Autodesk Fusion 360 part; units mm, degrees
(part 4 of 5)
equation "d178 = ( 7.087 / 2 ) * 1 mm + 2 mm"
equation "d179 = ( 7.087 / 2 ) * 1 mm + 2 mm"
equation "d208 = ( 36.1 / 2 ) * 1 mm"
equation "d215 = ( 4.85 / 2 ) * 1 mm + 2 mm"
equation "d216 = ( 4.85 / 2 ) * 1 mm + 2 mm"
equation "d221 = ( 4.85 / 2 ) * 1 mm + 2 mm"
equation "d222 = ( 4.85 / 2 ) * 1 mm + 2 mm"
equation "d230 = ( 36.1 / 2 ) * 1 mm"
equation "d251 = ( 11.15 / 2 ) * 1 mm"
equation "d266 = ( 11.15 / 2 ) * 1 mm"

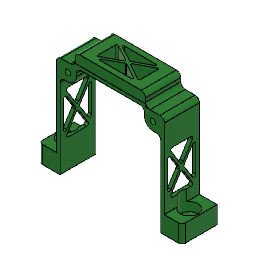
design "TM Front Holder"
Autodesk Fusion 360 part; units mm, degrees
sketch "Sketch1" plane through (0, 0, 0) normal (0, 0, 1) x (1, 0, 0)
  line L0 (28.55, 26.275) -> (30.55, 26.275)
  line L1 (30.55, 26.275) -> (30.55, -30.825)
  line L2 (30.55, -30.825) -> (28.55, -30.825)
  line L3 (28.55, -30.825) -> (28.55, 26.275)
  line L4 (-28.55, -30.825) -> (-30.55, -30.825)
  line L5 (-28.55, 26.275) -> (-28.55, -30.825)
  line L6 (-30.55, -30.825) -> (-30.55, 26.275)
  line L7 (-30.55, 26.275) -> (-28.55, 26.275)
  line L8 (-30.55, 26.275) -> (30.55, 26.275)
  line L9 (30.55, 26.275) -> (30.55, 28.275)
  line L10 (30.55, 28.275) -> (-30.55, 28.275)
  line L11 (-30.55, 28.275) -> (-30.55, 26.275)
  dimension "d1" = 2
  dimension "d4" = 26.275
  dimension "d5" = 2
  dimension "d7" = 57.1
  dimension "d8" = 28.55
  dimension "d9" = 2
  dimension "d99" = 59.1
  constraint horizontal L0
  constraint vertical L1
  constraint horizontal L2
  constraint vertical L3
  constraint horizontal L7
  constraint vertical L5
  constraint horizontal L4
  constraint vertical L6
  constraint horizontal L2.end L4.start
  constraint horizontal L8
  constraint vertical L9
  constraint horizontal L10
  constraint vertical L11
  constraint vertical L0.end L9.end
  measures "d1" distance of L1 L3
  measures "d4" distance of origin L0
  measures "d5" distance of L5 L6
  measures "d7" distance of L3 L5
  measures "d8" distance of origin L5
  measures "d9" distance of L8 L10
  measures "d99" distance of L2 L10
extrude "Extrude1" add sketch "Sketch1" along normal blind 20
sketch "Sketch2" plane through (0, 0, 20) normal (0, 0, 1) x (-1, 0, 0)
  line L0 (-30.55, 30.825) -> (-30.55, -28.275)
  line L1 (-30.55, -28.275) -> (30.55, -28.275)
  line L2 (30.55, -28.275) -> (30.55, 30.825)
  line L3 (30.55, 30.825) -> (28.55, 30.825)
  line L4 (28.55, 30.825) -> (28.55, -26.275)
  line L5 (28.55, -26.275) -> (-28.55, -26.275)
  line L6 (-28.55, -26.275) -> (-28.55, 30.825)
  line L7 (-28.55, 30.825) -> (-30.55, 30.825)
  line L8 (-30.55, 30.825) -> (-40.55, 30.825)
  line L9 (-40.55, 30.825) -> (-40.55, 28.325)
  line L10 (-40.55, 28.325) -> (-30.55, 28.325)
  line L11 (-30.55, 28.325) -> (-30.55, 30.825)
  line L12 (30.55, 30.825) -> (40.55, 30.825)
  line L13 (40.55, 30.825) -> (40.55, 28.325)
  line L14 (40.55, 28.325) -> (30.55, 28.325)
  line L15 (30.55, 28.325) -> (30.55, 30.825)
  dimension "d12" = 2.5
  dimension "d13" = 10
  dimension "d14" = 2.5
  dimension "d15" = 10
  constraint horizontal L8
  constraint vertical L9
  constraint horizontal L10
  constraint vertical L11
  constraint coincident L0.start L7.end
  constraint horizontal L12
  constraint vertical L13
  constraint horizontal L14
  constraint vertical L15
  constraint coincident L2.end L3.start
  measures "d12" distance of L8 L10
  measures "d13" distance of L9 L11
  measures "d14" distance of L12 L14
  measures "d15" distance of L13 L15
extrude "Extrude2" add sketch "Sketch2" against normal blind 20 contours L0 L8 L9 L10 L11 | L2 L12 L13 L14 L15
sketch "Sketch5" plane through (0, 28.275, 0) normal (0, 1, 0) x (-1, 0, 0)
  line L0 (-30.55, 0) -> (30.55, 0)
  line L1 (30.55, 0) -> (30.55, 20)
  line L2 (30.55, 20) -> (-30.55, 20)
  line L3 (-30.55, 20) -> (-30.55, 0)
  line L4 (-20, 20) -> (20, 20)
  line L5 (20, 20) -> (20, 0)
  line L6 (20, 0) -> (-20, 0)
  line L7 (-20, 0) -> (-20, 20)
  dimension "d32" = 40
  dimension "d96" = 20
  constraint horizontal L4
  constraint vertical L5
  constraint horizontal L6
  constraint vertical L7
  constraint coincident L0 L5.end
  constraint coincident L2 L4.start
  measures "d32" distance of L5 L7
  measures "d96" distance of origin L7
extrude "Extrude4" add sketch "Sketch5" along normal blind 10 contours L0 L2 L4 L5 L6 L7
sketch "Sketch6" plane through (0, 0, 0) normal (0, 0, -1) x (1, 0, 0)
  line L0 (20, -38.275) -> (20, -28.275)
  line L1 (-30.55, -28.275) -> (-20, -28.275)
  line L2 (30.55, -28.275) -> (30.55, 28.325)
  line L3 (30.55, 28.325) -> (40.55, 28.325)
  line L4 (40.55, 30.825) -> (28.55, 30.825)
  line L5 (28.55, 30.825) -> (28.55, -26.275)
  line L6 (28.55, -26.275) -> (-28.55, -26.275)
  line L7 (-28.55, -26.275) -> (-28.55, 30.825)
  line L8 (-28.55, 30.825) -> (-40.55, 30.825)
  line L9 (-40.55, 28.325) -> (-30.55, 28.325)
  line L10 (-30.55, 28.325) -> (-30.55, -28.275)
  line L11 (-20, -28.275) -> (-20, -38.275)
  line L12 (-20, -38.275) -> (20, -38.275)
  line L13 (-28.55, -26.275) -> (-19.3, -26.275)
  line L14 (-19.3, -23.775) -> (-19.3, -22.025)
  line L15 (-24.3, -17.025) -> (-26.05, -17.025)
  line L16 (-28.55, -17.025) -> (-28.55, -26.275)
  line L17 (28.55, -26.275) -> (19.3, -26.275)
  line L18 (19.3, -23.775) -> (19.3, -22.025)
  line L19 (24.3, -17.025) -> (26.05, -17.025)
  line L20 (28.55, -17.025) -> (28.55, -26.275)
  arc A0 (-19.3, -22.025) -> (-24.3, -17.025) centre (-24.3, -22.025) ccw
  arc A1 (24.3, -17.025) -> (19.3, -22.025) centre (24.3, -22.025) ccw
  line L21 (28.55, -14.525) -> (28.55, -10)
  line L22 (-28.55, -14.525) -> (-28.55, -10)
  arc A2 (26.05, -17.025) -> (28.55, -14.525) centre (26.05, -14.525) ccw
  arc A3 (-28.55, -14.525) -> (-26.05, -17.025) centre (-26.05, -14.525) ccw
  line L23 (16.8, -26.275) -> (13, -26.275)
  line L24 (-16.8, -26.275) -> (-13, -26.275)
  arc A4 (16.8, -26.275) -> (19.3, -23.775) centre (16.8, -23.775) ccw
  arc A5 (-19.3, -23.775) -> (-16.8, -26.275) centre (-16.8, -23.775) ccw
  line L25 (20, -28.275) -> (30.55, -28.275)
  line L26 (-40.55, 30.825) -> (-40.55, 28.325)
  line L27 (40.55, 28.325) -> (40.55, 30.825)
  dimension "d38" = 9.25
  dimension "d39" = 9.25
  dimension "d40" = 9.25
  dimension "d41" = 9.25
  dimension "d42" = 5
  dimension "d43" = 5
  dimension "d44" = 2.5
  dimension "d45" = 2.5
  dimension "d46" = 2.5
  dimension "d47" = 2.5
  constraint horizontal L13
  constraint vertical L14
  constraint horizontal L15
  constraint vertical L16
  constraint coincident L6.end L7.start
  constraint horizontal L17
  constraint vertical L18
  constraint horizontal L19
  constraint vertical L20
  constraint coincident L5.end L6.start
  constraint tangent L15 A0
  constraint tangent L14 A0
  constraint tangent L19 A1
  constraint tangent L18 A1
  constraint coincident L5 L21.end
  constraint coincident L7 L22.end
  constraint coincident L20.start L19
  constraint coincident L20.start L21
  constraint tangent L19 A2
  constraint tangent L21 A2
  constraint coincident L16.start L22
  constraint coincident L16.start L15
  constraint tangent L22 A3
  constraint tangent L15 A3
  constraint coincident L6 L23.end
  constraint coincident L6 L24.end
  constraint coincident L17.end L23
  constraint coincident L17.end L18
  constraint tangent L23 A4
  constraint tangent L18 A4
  constraint coincident L13.end L24
  constraint coincident L13.end L14
  constraint tangent L24 A5
  constraint tangent L14 A5
  measures "d38" distance of L14 L16
  measures "d39" distance of L13 L15
  measures "d40" distance of L18 L20
  measures "d41" distance of L17 L19
  measures "d42" radius of A0
  measures "d43" radius of A1
  measures "d44" radius of A2
  measures "d45" radius of A3
  measures "d46" radius of A4
  measures "d47" radius of A5
extrude "Extrude5" add sketch "Sketch6" against normal blind 20 contours L5 L6 L17 L18 L19 L20 A1 A2 A4 | L6 L7 L13 L14 L15 L16 A0 A3 A5
sketch "Sketch7" plane through (0, 0, 20) normal (0, 0, 1) x (-1, 0, 0)
  line L0 (-30.55, -28.275) -> (-20, -28.275)
  line L1 (-20, -28.275) -> (20, -28.275)
  line L2 (30.55, -28.275) -> (30.55, 28.325)
  line L3 (30.55, 28.325) -> (40.55, 28.325)
  line L4 (40.55, 28.325) -> (40.55, 30.825)
  line L5 (40.55, 30.825) -> (28.55, 30.825)
  line L6 (28.55, 30.825) -> (28.55, -14.525)
  arc A0 (26.05, -17.025) -> (28.55, -14.525) centre (26.05, -14.525) ccw
  line L7 (26.05, -17.025) -> (24.3, -17.025)
  arc A1 (24.3, -17.025) -> (19.3, -22.025) centre (24.3, -22.025) ccw
  line L8 (19.3, -22.025) -> (19.3, -23.775)
  arc A2 (16.8, -26.275) -> (19.3, -23.775) centre (16.8, -23.775) ccw
  line L9 (16.8, -26.275) -> (-16.8, -26.275)
  arc A3 (-19.3, -23.775) -> (-16.8, -26.275) centre (-16.8, -23.775) ccw
  line L10 (-19.3, -23.775) -> (-19.3, -22.025)
  arc A4 (-19.3, -22.025) -> (-24.3, -17.025) centre (-24.3, -22.025) ccw
  line L11 (-24.3, -17.025) -> (-26.05, -17.025)
  arc A5 (-28.55, -14.525) -> (-26.05, -17.025) centre (-26.05, -14.525) ccw
  line L12 (-28.55, -14.525) -> (-28.55, 30.825)
  line L13 (-28.55, 30.825) -> (-40.55, 30.825)
  line L14 (-40.55, 30.825) -> (-40.55, 28.325)
  line L15 (-40.55, 28.325) -> (-30.55, 28.325)
  line L16 (-30.55, 28.325) -> (-30.55, -28.275)
  line L17 (20, -28.275) -> (30.55, -28.275)
  point P0 (24.05, -21.775)
  point P1 (-24.05, -21.775)
  dimension "d52" = 6.5
  dimension "d54" = 6.5
  constraint horizontal P0 P1
  measures "d52" distance of L2 P0
  measures "d54" distance of L16 P1
hole "Hole2" at (-24.05, 21.775, 20) at (24.05, 21.775, 20) direction (0, 0, -1) diameter 3 end through all
sketch "Sketch9" plane through (0, 38.275, 0) normal (0, 1, 0) x (-1, 0, 0)
  line L0 (-20, 0) -> (20, 0)
  line L1 (20, 20) -> (-20, 20)
  line L2 (-9.0392, 17) -> (9.0392, 17)
  line L3 (-9.0392, 3) -> (9.0392, 3)
  line L4 (-12, 15.1577) -> (-12, 4.8423)
  line L5 (12, 15.1577) -> (12, 4.8399)
  line L6 (-9.2786, 3.9389) -> (-0.2394, 8.8694)
  line L7 (-11.2606, 4.4033) -> (-1.8047, 9.5611)
  line L8 (-1.8047, 10.4389) -> (-11.2606, 15.5967)
  line L9 (11.2606, 15.5967) -> (1.7742, 10.4223)
  line L10 (-9.2786, 16.0611) -> (-0.2394, 11.1306)
  line L11 (0.2394, 11.1306) -> (9.2786, 16.0611)
  line L12 (0.2394, 8.8694) -> (9.2786, 3.9389)
  line L13 (1.7753, 9.5438) -> (11.2617, 4.4003)
  arc A0 (-11.2606, 15.5967) -> (-12, 15.1577) centre (-11.5, 15.1577) ccw
  arc A1 (-1.8047, 9.5611) -> (-1.8047, 10.4389) centre (-2.0442, 10) ccw
  arc A2 (-12, 4.8423) -> (-11.2606, 4.4033) centre (-11.5, 4.8423) ccw
  arc A3 (-9.2786, 3.9389) -> (-9.0392, 3) centre (-9.0392, 3.5) ccw
  arc A4 (0.2394, 8.8694) -> (-0.2394, 8.8694) centre (0, 8.4305) ccw
  arc A5 (9.0392, 3) -> (9.2786, 3.9389) centre (9.0392, 3.5) ccw
  arc A6 (11.2617, 4.4003) -> (12, 4.8399) centre (11.5, 4.8399) ccw
  arc A7 (1.7742, 10.4223) -> (1.7753, 9.5438) centre (2.0137, 9.9834) ccw
  arc A8 (12, 15.1577) -> (11.2606, 15.5967) centre (11.5, 15.1577) ccw
  arc A9 (9.2786, 16.0611) -> (9.0392, 17) centre (9.0392, 16.5) ccw
  arc A10 (-9.0392, 17) -> (-9.2786, 16.0611) centre (-9.0392, 16.5) ccw
  arc A11 (-0.2394, 11.1306) -> (0.2394, 11.1306) centre (0, 11.5695) ccw
  line L14 (20, 0) -> (20, 20)
  line L15 (-20, 20) -> (-20, 0)
  point P0 (11, 17)
  point P1 (12, 16)
  point P2 (0, 10)
  dimension "d60" = 11
  dimension "d61" = 6
  dimension "d62" = 0.5
  constraint horizontal L3
  constraint vertical L4
  constraint vertical L5
  constraint parallel L7 L9
  constraint tangent L4 A0
  constraint tangent L8 A0
  constraint tangent L8 A1
  constraint tangent L7 A1
  constraint equal A0 A1
  constraint tangent L4 A2
  constraint tangent L7 A2
  constraint equal A0 A2
  constraint tangent L3 A3
  constraint tangent L6 A3
  constraint equal A0 A3
  constraint tangent L12 A4
  constraint tangent L6 A4
  constraint equal A0 A4
  constraint tangent L12 A5
  constraint tangent L3 A5
  constraint equal A0 A5
  constraint tangent L13 A6
  constraint tangent L5 A6
  constraint equal A0 A6
  constraint tangent L9 A7
  constraint tangent L13 A7
  constraint equal A0 A7
  constraint coincident P1 L5
  constraint coincident P1 L9
  constraint tangent L5 A8
  constraint tangent L9 A8
  constraint equal A0 A8
  constraint coincident P0 L11
  constraint tangent L11 A9
  constraint tangent L2 A9
  constraint equal A0 A9
  constraint tangent L2 A10
  constraint tangent L10 A10
  constraint equal A0 A10
  constraint tangent L11 A11
  constraint tangent L10 A11
  constraint equal A0 A11
  measures "d60" horizontal distance of P0 P2
  measures "d61" vertical distance of P1 P2
  measures "d62" radius of A0
extrude "Extrude7" cut sketch "Sketch9" against normal blind 15 contours L2 L10 L11 A9 A10 A11 | L3 L6 L12 A3 A4 A5 | L4 L7 L8 A0 A1 A2 | L5 L9 L13 A6 A7 A8
sketch "Sketch10" plane through (-30.55, 0, 0) normal (-1, 0, 0) x (0, -1, 0)
  line L0 (-28.275, 0) -> (28.325, 0)
  line L1 (28.325, 0) -> (28.325, 20)
  line L2 (28.325, 20) -> (-28.275, 20)
  line L3 (-9.975, 15.25) -> (-9.975, 4.85)
  line L4 (14.525, 15.25) -> (14.525, 4.85)
  line L5 (-28.275, 20) -> (-28.275, 0)
  line L6 (-5.2906, 18) -> (9.8406, 18)
  line L7 (-5.2906, 2) -> (9.8406, 2)
  line L8 (-5.8274, 3.8437) -> (1.7382, 8.6576)
  line L9 (2.8118, 8.6576) -> (10.3774, 3.8437)
  line L10 (12.9967, 4.0009) -> (4.6396, 9.2009)
  line L11 (4.6396, 10.8991) -> (12.9967, 16.0991)
  line L12 (10.3774, 16.1563) -> (2.8118, 11.3424)
  line L13 (1.7382, 11.3424) -> (-5.8274, 16.1563)
  line L14 (-8.4467, 16.0991) -> (-0.0896, 10.8991)
  line L15 (-0.0896, 9.2009) -> (-8.4467, 4.0009)
  arc A0 (-8.4467, 16.0991) -> (-9.975, 15.25) centre (-8.975, 15.25) ccw
  arc A1 (-9.975, 4.85) -> (-8.4467, 4.0009) centre (-8.975, 4.85) ccw
  arc A2 (-0.0896, 9.2009) -> (-0.0896, 10.8991) centre (-0.6179, 10.05) ccw
  arc A3 (2.8118, 8.6576) -> (1.7382, 8.6576) centre (2.275, 7.8139) ccw
  arc A4 (9.8406, 2) -> (10.3774, 3.8437) centre (9.8406, 3) ccw
  arc A5 (-5.8274, 3.8437) -> (-5.2906, 2) centre (-5.2906, 3) ccw
  arc A6 (12.9967, 4.0009) -> (14.525, 4.85) centre (13.525, 4.85) ccw
  arc A7 (14.525, 15.25) -> (12.9967, 16.0991) centre (13.525, 15.25) ccw
  arc A8 (10.3774, 16.1563) -> (9.8406, 18) centre (9.8406, 17) ccw
  arc A9 (-5.2906, 18) -> (-5.8274, 16.1563) centre (-5.2906, 17) ccw
  arc A10 (1.7382, 11.3424) -> (2.8118, 11.3424) centre (2.275, 12.1861) ccw
  arc A11 (4.6396, 10.8991) -> (4.6396, 9.2009) centre (5.1679, 10.05) ccw
  line L16 (-28.275, 20) -> (-28.275, 0)
  point P0 (-9.975, 17.05)
  point P1 (-9.975, 3.05)
  point P2 (14.525, 17.05)
  point P3 (14.525, 3.05)
  point P4 (-8.725, 18)
  point P5 (13.275, 18)
  point P6 (-8.725, 2)
  point P7 (13.275, 2)
  point P8 (2.275, 10.05)
  dimension "d79" = 2
  dimension "d80" = 2
  dimension "d81" = 11
  dimension "d82" = 7
  dimension "d83" = 22
  dimension "d84" = 22
  dimension "d85" = 14
  dimension "d86" = 14
  dimension "d88" = 3.05
  dimension "d89" = 1
  dimension "d100" = 24.5
  dimension "d101" = 5.7857
  constraint perpendicular L2 L3
  constraint vertical L4
  constraint horizontal L6
  constraint perpendicular L3 L7
  constraint horizontal P0 P2
  constraint vertical P4 P6
  constraint coincident P0 L14
  constraint coincident P0 L3
  constraint tangent L14 A0
  constraint tangent L3 A0
  constraint coincident P1 L3
  constraint coincident P1 L15
  constraint tangent L3 A1
  constraint tangent L15 A1
  constraint equal A0 A1
  constraint tangent L15 A2
  constraint tangent L14 A2
  constraint equal A0 A2
  constraint tangent L8 A3
  constraint tangent L9 A3
  constraint equal A0 A3
  constraint coincident P7 L9
  constraint coincident P7 L7
  constraint tangent L9 A4
  constraint tangent L7 A4
  constraint equal A0 A4
  constraint coincident P6 L7
  constraint coincident P6 L8
  constraint tangent L7 A5
  constraint tangent L8 A5
  constraint equal A0 A5
  constraint coincident P3 L10
  constraint coincident P3 L4
  constraint tangent L10 A6
  constraint tangent L4 A6
  constraint equal A0 A6
  constraint coincident P2 L4
  constraint coincident P2 L11
  constraint tangent L4 A7
  constraint tangent L11 A7
  constraint equal A0 A7
  constraint coincident P5 L12
  constraint coincident P5 L6
  constraint tangent L12 A8
  constraint tangent L6 A8
  constraint equal A0 A8
  constraint coincident P4 L13
  constraint coincident P4 L6
  constraint tangent L13 A9
  constraint tangent L6 A9
  constraint equal A0 A9
  constraint tangent L13 A10
  constraint equal A0 A10
  constraint tangent L10 A11
  constraint tangent L11 A11
  constraint equal A0 A11
  constraint horizontal A0.centre A7.centre
  constraint horizontal A1.centre A6.centre
  constraint vertical A5.centre A9.centre
  constraint vertical A4.centre A8.centre
  constraint horizontal P8 A2.centre
  constraint vertical P8 A3.centre
  measures "d79" distance of L2 L6
  measures "d80" distance of L0 L7
  measures "d81" horizontal distance of P5 P8
  measures "d82" vertical distance of P2 P8
  measures "d83" distance of P4 P5
  measures "d84" distance of P6 P7
  measures "d85" distance of P2 P3
  measures "d86" distance of P0 P1
  measures "d88" distance of L0 P3
  measures "d89" radius of A0
  measures "d100" distance of L3 L4
  measures "d101" horizontal distance of A2.centre A11.centre
extrude "Extrude8" cut sketch "Sketch10" against normal blind 65 contours L3 L14 L15 A0 A1 A2 | L4 L10 L11 A6 A7 A11 | L6 L12 L13 A8 A9 A10 | L7 L8 L9 A3 A4 A5
extrude "Extrude9" cut 2 faces at (27.0333, 28.275, 6.6667) (-23.5167, 28.275, 13.3333) along direction (0, -1, 0) blind 1.55
extrude "Extrude10" cut 1 faces at (-17.3333, 38.275, 11.7192) along direction (0, -1, 0) blind 4.5
fillet "Fillet4" radius 2.5 6 edges at (-20, 26.725, 10) (-20, 33.775, 10) (-30.55, 26.725, 10) (20, 33.775, 10) (20, 26.725, 10) (30.55, 26.725, 10)
fillet "Fillet5" radius 2 2 edges at (-40.55, -29.575, 20) (40.55, -29.575, 20)
extrude "Extrude11" cut 2 faces at (-32.55, -30.825, 12.6667) (32.55, -30.825, 12.6667) along direction (0, 1, 0) blind 0.05
extrude "Extrude12" add 2 faces at (33.8833, -28.325, 12.6667) (-33.8833, -28.325, 12.6667) along direction (0, 1, 0) blind 7.55
sketch "Sketch11" plane through (0, -20.775, 0) normal (0, 1, 0) x (-1, 0, 0)
  arc A0 (-38.55, 20) -> (-40.55, 18) centre (-38.55, 18) ccw
  line L0 (-40.55, 18) -> (-40.55, 0)
  line L1 (-40.55, 0) -> (-30.55, 0)
  line L2 (-30.55, 0) -> (-30.55, 20)
  line L3 (-30.55, 20) -> (-38.55, 20)
  point P0 (-34.75, 10)
  point P1 (34.75, 10)
  dimension "d112" = 69.5
  dimension "d113" = 5.8
  dimension "d114" = 10
  constraint horizontal P0 P1
  measures "d112" distance of P0 P1
  measures "d113" distance of L0 P0
  measures "d114" distance of L3 P0
hole "Hole3" at (34.75, -20.775, 10) at (-34.75, -20.775, 10) direction (0, -1, 0) diameter 5.3 end through all counterbore diameter 10 counterbore depth 5
sketch "Sketch12" plane through (0, -20.775, 0) normal (0, 1, 0) x (-1, 0, 0)
  arc A0 (-30.55, 12.7129) -> (-30.55, 7.2871) centre (-34.75, 10) ccw
  line L0 (-30.55, 12.7129) -> (-30.55, 20)
  line L1 (-30.55, 20) -> (-38.55, 20)
  arc A1 (-38.55, 20) -> (-40.55, 18) centre (-38.55, 18) ccw
  line L2 (-40.55, 18) -> (-40.55, 0)
  line L3 (-40.55, 0) -> (-30.55, 0)
  line L4 (-30.55, 0) -> (-30.55, 7.2871)
  circle A2 centre (-34.75, 10) radius 5
  circle A3 centre (34.75, 10) radius 5
  dimension "d119" = 10
  dimension "d120" = 10
  dimension "d121" = 69.5
  constraint concentric A0 A2
  constraint horizontal A0.centre A3.centre
  measures "d119" diameter of A2
  measures "d120" diameter of A3
  measures "d121" distance of A0.centre A3.centre
extrude "Extrude13" cut sketch "Sketch12" along normal blind 7 contours A0 A2 | A3
equation "d4 = ( 52.55 / 2 ) * 1 mm"
equation "d8 = ( 57.1 / 2 ) * 1 mm"
equation "d88 = ( ( 20.1 - 14 ) / 2 ) * 1 mm"
equation "d99 = 57.55 mm + 1.55 mm"
equation "d110 = 10 mm - 2.45 mm"

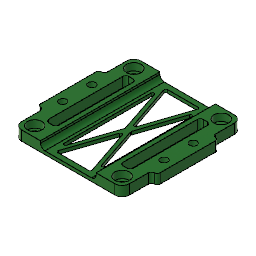
design "LGR RM Carriage Bracket (Defensemen)"
Autodesk Fusion 360 part; units mm, degrees
sketch "Sketch1" plane through (0, 0, 0) normal (0, 0, 1) x (1, 0, 0)
  line L0 (-41, 41) -> (41, 41)
  line L1 (41, 41) -> (41, -41)
  line L2 (41, -41) -> (-41, -41)
  line L3 (-41, -41) -> (-41, 41)
  dimension "d1" = 82
  dimension "d2" = 82
  dimension "d3" = 41
  dimension "d4" = 41
  constraint horizontal L0
  constraint vertical L1
  constraint horizontal L2
  constraint vertical L3
  measures "d1" distance of L1 L3
  measures "d2" distance of L0 L2
  measures "d3" distance of origin L1
  measures "d4" distance of origin L0
extrude "Extrude1" add sketch "Sketch1" along normal blind 6.5
sketch "Sketch2" plane through (0, 0, 6.5) normal (0, 0, 1) x (-1, 0, 0)
  line L0 (41, 41) -> (-41, 41)
  line L1 (-41, 41) -> (-41, -41)
  line L2 (-41, -41) -> (41, -41)
  line L3 (41, -41) -> (41, 41)
  point P0 (34, -30)
  point P1 (-34, -30)
  point P2 (-34, 30)
  point P3 (34, 30)
  dimension "d7" = 68
  dimension "d8" = 60
  dimension "d9" = 7
  dimension "d10" = 11
  constraint horizontal P0 P1
  constraint vertical P1 P2
  constraint horizontal P2 P3
  constraint vertical P0 P3
  measures "d7" distance of P0 P1
  measures "d8" distance of P1 P2
  measures "d9" distance of L1 P1
  measures "d10" distance of L2 P1
hole "Hole1" at (-34, 30, 6.5) at (34, 30, 6.5) at (34, -30, 6.5) at (-34, -30, 6.5) direction (0, 0, -1) diameter 5.5 depth 10 tip angle 180 counterbore diameter 10 counterbore depth 5
sketch "Sketch3" plane through (0, 0, 6.5) normal (0, 0, 1) x (-1, 0, 0)
  circle A0 centre (-34, 30) radius 5
  circle A1 centre (34, -30) radius 5
  circle A2 centre (-34, -30) radius 5
  circle A3 centre (34, 30) radius 5
  line L0 (41, 41) -> (-41, 41)
  line L1 (-41, 41) -> (-41, -41)
  line L2 (-41, -41) -> (41, -41)
  line L3 (41, -41) -> (41, 41)
  line L4 (41, -19.05) -> (-41, -19.05)
  line L5 (-41, -19.05) -> (-41, 19.05)
  line L6 (-41, 19.05) -> (41, 19.05)
  line L7 (41, 19.05) -> (41, -19.05)
  dimension "d16" = 38.1
  dimension "d17" = 19.05
  constraint horizontal L4
  constraint vertical L5
  constraint horizontal L6
  constraint vertical L7
  constraint coincident L1 L5.end
  constraint coincident L3 L4.start
  measures "d16" distance of L4 L6
  measures "d17" distance of origin L6
extrude "Extrude2" cut sketch "Sketch3" against normal blind 4.5 contours L1 L3 L4 L5 L6 L7
fillet "Fillet1" radius 3 2 edges at (0, 19.05, 2) (0, -19.05, 2)
sketch "Sketch4" plane through (0, 0, 6.5) normal (0, 0, 1) x (-1, 0, 0)
  line L0 (41, -19.05) -> (-41, -19.05)
  line L1 (-41, -19.05) -> (-41, -41)
  line L2 (-41, -41) -> (41, -41)
  line L3 (41, -41) -> (41, -19.05)
  circle A0 centre (34, -30) radius 5
  circle A1 centre (-34, -30) radius 5
  line L4 (41, 41) -> (-41, 41)
  line L5 (41, 19.05) -> (41, 41)
  point P0 (-10, -34.75)
  point P1 (10, -34.75)
  point P2 (-10, 34.75)
  point P3 (10, 34.75)
  point P4 (-5.7919, 53.9874)
  dimension "d23" = 6.25
  dimension "d24" = 6.25
  dimension "d25" = 20
  dimension "d26" = 31
  constraint vertical P0 P2
  constraint horizontal P2 P3
  constraint vertical P1 P3
  constraint horizontal P0 P1
  measures "d23" distance of P2 L4
  measures "d24" distance of L2 P0
  measures "d25" distance of P0 P1
  measures "d26" distance of P3 L5
hole "Hole2" at (10, 34.75, 6.5) at (-10, 34.75, 6.5) at (10, -34.75, 6.5) at (-10, -34.75, 6.5) direction (0, 0, -1) diameter 5 end through all
sketch "Sketch7" plane through (0, 0, 6.5) normal (0, 0, 1) x (-1, 0, 0)
  circle A0 centre (-10, 34.75) radius 2.5
  circle A1 centre (10, 34.75) radius 2.5
  line L0 (-41, 19.05) -> (41, 19.05)
  line L1 (41, 19.05) -> (41, 41)
  line L2 (41, 41) -> (-41, 41)
  line L3 (-41, 41) -> (-41, 19.05)
  circle A2 centre (34, 30) radius 5
  circle A3 centre (-34, 30) radius 5
  line L4 (25.5, 22.05) -> (-25.5, 22.05)
  line L5 (-27.5, 24.05) -> (-27.5, 27.05)
  line L6 (-25.5, 29.05) -> (25.5, 29.05)
  line L7 (27.5, 27.05) -> (27.5, 24.05)
  line L8 (25.5, -29.05) -> (-25.5, -29.05)
  line L9 (-27.5, -27.05) -> (-27.5, -24.05)
  line L10 (-25.5, -22.05) -> (25.5, -22.05)
  line L11 (27.5, -24.05) -> (27.5, -27.05)
  line L12 (41, -19.05) -> (-41, -19.05)
  line L13 (-41, -19.05) -> (-41, -41)
  arc A4 (25.5, -29.05) -> (27.5, -27.05) centre (25.5, -27.05) ccw
  arc A5 (27.5, -24.05) -> (25.5, -22.05) centre (25.5, -24.05) ccw
  arc A6 (-25.5, -22.05) -> (-27.5, -24.05) centre (-25.5, -24.05) ccw
  arc A7 (-27.5, -27.05) -> (-25.5, -29.05) centre (-25.5, -27.05) ccw
  arc A8 (25.5, 22.05) -> (27.5, 24.05) centre (25.5, 24.05) ccw
  arc A9 (27.5, 27.05) -> (25.5, 29.05) centre (25.5, 27.05) ccw
  arc A10 (-25.5, 29.05) -> (-27.5, 27.05) centre (-25.5, 27.05) ccw
  arc A11 (-27.5, 24.05) -> (-25.5, 22.05) centre (-25.5, 24.05) ccw
  dimension "d31" = 55
  dimension "d32" = 7
  dimension "d33" = 3
  dimension "d34" = 13.5
  dimension "d35" = 7
  dimension "d36" = 3
  dimension "d37" = 13.5
  dimension "d38" = 55
  dimension "d39" = 2
  constraint horizontal L4
  constraint vertical L5
  constraint horizontal L6
  constraint vertical L7
  constraint horizontal L8
  constraint vertical L9
  constraint horizontal L10
  constraint vertical L11
  constraint tangent L8 A4
  constraint tangent L11 A4
  constraint tangent L11 A5
  constraint tangent L10 A5
  constraint equal A4 A5
  constraint tangent L10 A6
  constraint tangent L9 A6
  constraint equal A4 A6
  constraint tangent L9 A7
  constraint tangent L8 A7
  constraint equal A4 A7
  constraint tangent L4 A8
  constraint tangent L7 A8
  constraint equal A4 A8
  constraint tangent L7 A9
  constraint tangent L6 A9
  constraint equal A4 A9
  constraint tangent L6 A10
  constraint tangent L5 A10
  constraint equal A4 A10
  constraint tangent L5 A11
  constraint tangent L4 A11
  constraint equal A4 A11
  measures "d31" distance of L5 L7
  measures "d32" distance of L4 L6
  measures "d33" distance of L0 L4
  measures "d34" distance of L1 L7
  measures "d35" distance of L8 L10
  measures "d36" distance of L10 L12
  measures "d37" distance of L9 L13
  measures "d38" distance of L9 L11
  measures "d39" radius of A4
extrude "Extrude3" cut sketch "Sketch7" against normal blind 6.5 contours L4 L5 L6 L7 A8 A9 A10 A11 | L8 L9 L10 L11 A4 A5 A6 A7
ref_plane "WorkPlane1" through (0, 0, 6.5) normal (0, 0, -1) x (-1, 0, 0)
sketch "Sketch9" plane through (0, 0, 6.5) normal (0, 0, -1) x (-1, 0, 0)
  line L0 (41, 41) -> (21, 41)
  line L1 (21, 41) -> (21, 37)
  line L2 (21, 37) -> (41, 37)
  line L3 (41, 37) -> (41, 41)
  line L4 (-21, 41) -> (-41, 41)
  line L5 (-41, 41) -> (-41, 37)
  line L6 (-41, 37) -> (-21, 37)
  line L7 (-21, 37) -> (-21, 41)
  line L8 (41, -37) -> (21, -37)
  line L9 (21, -37) -> (21, -41)
  line L10 (21, -41) -> (41, -41)
  line L11 (41, -41) -> (41, -37)
  line L12 (-41, -41) -> (-21, -41)
  line L13 (-21, -41) -> (-21, -37)
  line L14 (-21, -37) -> (-41, -37)
  line L15 (-41, -37) -> (-41, -41)
  point P0 (41, 41)
  dimension "d59" = 82
  dimension "d60" = 82
  dimension "d61" = 4
  dimension "d62" = 20
  dimension "d63" = 20
  dimension "d64" = 4
  dimension "d65" = 20
  dimension "d66" = 20
  dimension "d67" = 4
  dimension "d68" = 4
  constraint horizontal L0
  constraint vertical L1
  constraint horizontal L2
  constraint vertical L3
  constraint horizontal L4
  constraint vertical L5
  constraint horizontal L6
  constraint vertical L7
  constraint horizontal L8
  constraint vertical L9
  constraint horizontal L10
  constraint vertical L11
  constraint horizontal L12
  constraint vertical L13
  constraint horizontal L14
  constraint vertical L15
  constraint vertical P0 L10.end
  constraint horizontal P0 L4.end
  constraint vertical L4.end L12.start
  constraint horizontal L10.end L12.start
  constraint vertical P0 L0.start
  constraint horizontal L0.end P0
  measures "d59" distance of L3 L5
  measures "d60" distance of L0 L10
  measures "d61" distance of L0 L2
  measures "d62" distance of L1 L3
  measures "d63" distance of L5 L7
  measures "d64" distance of L4 L6
  measures "d65" distance of L13 L15
  measures "d66" distance of L9 L11
  measures "d67" distance of L8 L10
  measures "d68" distance of L12 L14
extrude "Extrude5" cut sketch "Sketch9" along normal blind 6.5
fillet "Fillet2" radius 5 4 edges at (-41, 37, 3.25) (41, 37, 3.25) (41, -37, 3.25) (-41, -37, 3.25)
fillet "Fillet3" radius 2 8 edges at (-21, -41, 3.25) (-21, -37, 3.25) (21, -37, 3.25) (21, -41, 3.25) (21, 37, 3.25) (21, 41, 3.25) (-21, 41, 3.25) (-21, 37, 3.25)
sketch "Sketch10" plane through (0, 0, 2) normal (0, 0, 1) x (-1, 0, 0)
  line L0 (41, 16.05) -> (-41, 16.05)
  line L1 (-41, 16.05) -> (-41, -16.05)
  line L2 (-41, -16.05) -> (41, -16.05)
  line L3 (41, -16.05) -> (41, 16.05)
  line L4 (29.8377, -14) -> (-29.8377, -14)
  line L5 (29.8377, 14) -> (-29.8377, 14)
  line L6 (37.5, -10.6064) -> (37.5, 10.6064)
  line L7 (-37.5, -10.6064) -> (-37.5, 10.6064)
  line L8 (41, -19.05) -> (-41, -19.05)
  line L9 (30.154, 12.0513) -> (0.3162, 2.1054)
  line L10 (-0.3162, 2.1054) -> (-30.154, 12.0513)
  line L11 (-36.1798, 11.5537) -> (-4.8025, 0.9473)
  line L12 (-4.8025, -0.9473) -> (-36.1798, -11.5537)
  line L13 (-30.154, -12.0513) -> (-0.3162, -2.1054)
  line L14 (0.3162, -2.1054) -> (30.154, -12.0513)
  line L15 (36.1798, -11.5537) -> (4.8025, -0.9473)
  line L16 (4.8025, 0.9473) -> (36.1798, 11.5537)
  arc A0 (29.8377, -14) -> (30.154, -12.0513) centre (29.8377, -13) ccw
  arc A1 (0.3162, -2.1054) -> (-0.3162, -2.1054) centre (0, -3.0541) ccw
  arc A2 (-30.154, -12.0513) -> (-29.8377, -14) centre (-29.8377, -13) ccw
  arc A3 (-37.5, -10.6064) -> (-36.1798, -11.5537) centre (-36.5, -10.6064) ccw
  arc A4 (-36.1798, 11.5537) -> (-37.5, 10.6064) centre (-36.5, 10.6064) ccw
  arc A5 (-4.8025, -0.9473) -> (-4.8025, 0.9473) centre (-5.1228, 0) ccw
  arc A6 (-0.3162, 2.1054) -> (0.3162, 2.1054) centre (0, 3.0541) ccw
  arc A7 (-29.8377, 14) -> (-30.154, 12.0513) centre (-29.8377, 13) ccw
  arc A8 (30.154, 12.0513) -> (29.8377, 14) centre (29.8377, 13) ccw
  arc A9 (37.5, 10.6064) -> (36.1798, 11.5537) centre (36.5, 10.6064) ccw
  arc A10 (36.1798, -11.5537) -> (37.5, -10.6064) centre (36.5, -10.6064) ccw
  arc A11 (4.8025, 0.9473) -> (4.8025, -0.9473) centre (5.1228, 0) ccw
  point P0 (36, -14)
  point P1 (-36, -14)
  point P2 (-37.5, -12)
  point P3 (-37.5, 12)
  point P4 (0, -2)
  point P5 (-2, 0)
  point P6 (0, 2)
  point P7 (2, 0)
  dimension "d75" = 72
  dimension "d76" = 24
  dimension "d77" = 5
  dimension "d78" = 7.05
  dimension "d79" = 2.05
  dimension "d80" = 2.05
  dimension "d81" = 3.5
  dimension "d82" = 3.5
  dimension "d83" = 1
  constraint parallel L2 L4
  constraint perpendicular L3 L5
  constraint perpendicular L5 L6
  constraint perpendicular L4 L7
  constraint coincident P0 L4
  constraint coincident P0 L14
  constraint tangent L4 A0
  constraint tangent L14 A0
  constraint tangent L14 A1
  constraint tangent L13 A1
  constraint equal A0 A1
  constraint coincident P1 L13
  constraint coincident P1 L4
  constraint tangent L13 A2
  constraint tangent L4 A2
  constraint equal A0 A2
  constraint coincident P2 L12
  constraint coincident P2 L7
  constraint tangent L12 A3
  constraint tangent L7 A3
  constraint equal A0 A3
  constraint coincident P3 L7
  constraint coincident P3 L11
  constraint tangent L7 A4
  constraint tangent L11 A4
  constraint equal A0 A4
  constraint tangent L11 A5
  constraint tangent L12 A5
  constraint equal A0 A5
  constraint tangent L10 A6
  constraint tangent L9 A6
  constraint equal A0 A6
  constraint tangent L10 A7
  constraint tangent L5 A7
  constraint equal A0 A7
  constraint tangent L5 A8
  constraint tangent L9 A8
  constraint equal A0 A8
  constraint tangent L16 A9
  constraint tangent L6 A9
  constraint equal A0 A9
  constraint tangent L6 A10
  constraint tangent L15 A10
  constraint equal A0 A10
  constraint tangent L15 A11
  constraint tangent L16 A11
  constraint equal A0 A11
  measures "d75" distance of P0 P1
  measures "d76" distance of P2 P3
  measures "d77" distance of L1 P1
  measures "d78" distance of P2 L8
  measures "d79" distance of L2 L4
  measures "d80" distance of L0 L5
  measures "d81" distance of L1 L7
  measures "d82" distance of L3 L6
  measures "d83" radius of A0
extrude "Extrude6" cut sketch "Sketch10" against normal blind 2 contours L4 L13 L14 A0 A1 A2 | L5 L9 L10 A6 A7 A8 | L6 L15 L16 A9 A10 A11 | L7 L11 L12 A3 A4 A5
extrude "Extrude7" add 1 faces at (8.5, 16.6833, 0) along direction (0, 0, -1) blind 0.25
equation "d3 = ( 82 / 2 ) * 1 mm"
equation "d4 = ( 82 / 2 ) * 1 mm"
equation "d9 = ( ( 82 - 68 ) / 2 ) * 1 mm"
equation "d10 = ( ( 82 - 60 ) / 2 ) * 1 mm"
equation "d17 = ( 38.1 / 2 ) * 1 mm"
equation "d26 = ( ( 82 - 20 ) / 2 ) * 1 mm"
equation "d34 = ( ( 82 - 55 ) / 2 ) * 1 mm"
equation "d37 = ( ( 82 - 55 ) / 2 ) * 1 mm"
equation "d77 = ( ( 82 - 72 ) / 2 ) * 1 mm"
equation "d78 = ( ( 38.1 - 24 ) / 2 ) * 1 mm"

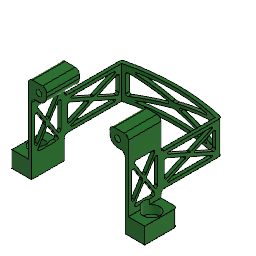
design "LGR RM Back Holder (Defensemen)"
Autodesk Fusion 360 part; units mm, degrees
sketch "Sketch1" plane through (0, 0, 0) normal (0, 0, 1) x (1, 0, 0)
  line L0 (-30.55, 55) -> (-28.55, 55)
  line L1 (-28.55, 55) -> (-28.55, 0)
  line L2 (-28.55, 0) -> (-30.55, 0)
  line L3 (-30.55, 0) -> (-30.55, 55)
  line L4 (28.55, 55) -> (30.55, 55)
  line L5 (30.55, 55) -> (30.55, 0)
  line L6 (30.55, 0) -> (28.55, 0)
  line L7 (28.55, 0) -> (28.55, 55)
  dimension "d1" = 55
  dimension "d2" = 55
  dimension "d3" = 2
  dimension "d4" = 2
  dimension "d5" = 57.1
  dimension "d6" = 28.55
  constraint horizontal L0
  constraint vertical L1
  constraint horizontal L2
  constraint vertical L3
  constraint horizontal L4
  constraint vertical L5
  constraint horizontal L6
  constraint vertical L7
  constraint horizontal L0.start L4.start
  constraint horizontal origin L1.end
  measures "d1" distance of L0 L2
  measures "d2" distance of L4 L6
  measures "d3" distance of L1 L3
  measures "d4" distance of L5 L7
  measures "d5" distance of L1 L7
  measures "d6" distance of origin L7
extrude "Extrude1" add sketch "Sketch1" along normal blind 20 makes body 1 at (-28.55, 36.6667, 6.6667) makes body 2 at (30.55, 36.6667, 6.6667)
sketch "Sketch3" plane through (0, 0, 20) normal (0, 0, 1) x (-1, 0, 0)
  line L0 (-28.55, 0) -> (-30.55, 0)
  line L1 (-30.55, 0) -> (-30.55, -55)
  line L2 (-30.55, -55) -> (-28.55, -55)
  line L3 (-28.55, -55) -> (-28.55, 0)
  arc A0 (-28.55, -55) -> (28.55, -55) centre (0, 53.299) ccw
  arc A1 (-30.55, -57) -> (30.55, -57) centre (0, 67.272) ccw
  line L4 (30.55, -57) -> (30.55, -55)
  line L5 (-30.55, -57) -> (-30.55, -55)
  line L6 (-28.55, -55) -> (-30.55, -55)
  line L7 (28.55, -55) -> (30.55, -55)
  point P0 (-28.55, -55)
  point P1 (28.55, -55)
  point P2 (0, -58.7)
  point P3 (0, -60.7)
  point P4 (30.55, -57)
  point P5 (-30.55, -57)
  point P6 (30.55, -55)
  point P7 (28.55, -55)
  dimension "d9" = 3.7
  dimension "d10" = 2
  dimension "d11" = 2
  dimension "d12" = 2
  constraint coincident P0 L2.end
  constraint coincident P2 A0
  constraint coincident P7 P1
  constraint vertical origin P2
  constraint vertical P2 P3
  constraint vertical L1.end P5
  constraint vertical P4 P6
  constraint coincident P3 A1
  constraint coincident P5 A1.start
  constraint coincident P4 A1.end
  constraint coincident P6 L4.end
  constraint coincident L1.end L2.start
  measures "d9" vertical distance of P0 P2
  measures "d10" distance of P2 P3
  measures "d11" distance of P4 P6
  measures "d12" distance of L1.end P5
extrude "Extrude2" add sketch "Sketch3" against normal blind 20 contours L2 A0 A1 L4 L5 L6 L7 bodies 1 2
sketch "Sketch4" plane through (30.55, 0, 0) normal (1, 0, 0) x (0, 1, 0)
  line L0 (0, 0) -> (57, 0)
  line L1 (57, 0) -> (57, 20)
  line L2 (57, 20) -> (0, 20)
  line L3 (0, 20) -> (0, 0)
  line L4 (0, 0) -> (20, 0)
  line L5 (20, 0) -> (20, -4)
  line L6 (20, -4) -> (0, -4)
  line L7 (0, -4) -> (0, 0)
  dimension "d15" = 4
  dimension "d16" = 20
  constraint horizontal L4
  constraint vertical L5
  constraint horizontal L6
  constraint vertical L7
  constraint coincident L0.start L3.end
  measures "d15" distance of L4 L6
  measures "d16" distance of L5 L7
extrude "Extrude3" add sketch "Sketch4" against normal blind 2 contours L0 L4 L5 L6 L7 bodies 1
sketch "Sketch5" plane through (-30.55, 0, 0) normal (-1, 0, 0) x (0, -1, 0)
  line L0 (-57, 0) -> (0, 0)
  line L1 (0, 0) -> (0, 20)
  line L2 (0, 20) -> (-57, 20)
  line L3 (-57, 20) -> (-57, 0)
  line L4 (0, 0) -> (-20, 0)
  line L5 (-20, 0) -> (-20, -4)
  line L6 (-20, -4) -> (0, -4)
  line L7 (0, -4) -> (0, 0)
  dimension "d19" = 4
  dimension "d20" = 20
  constraint horizontal L4
  constraint vertical L5
  constraint horizontal L6
  constraint vertical L7
  constraint coincident L0.end L1.start
  measures "d19" distance of L4 L6
  measures "d20" distance of L5 L7
extrude "Extrude4" add sketch "Sketch5" against normal blind 2 contours L0 L4 L5 L6 L7 bodies 1
sketch "Sketch6" plane through (0, 0, 0) normal (0, -1, 0) x (1, 0, 0)
  line L0 (30.55, -4) -> (30.55, 20)
  line L1 (30.55, 20) -> (28.55, 20)
  line L2 (28.55, 20) -> (28.55, -4)
  line L3 (28.55, -4) -> (30.55, -4)
  line L4 (28.55, -4) -> (40.55, -4)
  line L5 (40.55, -4) -> (40.55, -14)
  line L6 (40.55, -14) -> (28.55, -14)
  line L7 (28.55, -14) -> (28.55, -4)
  line L8 (-28.55, -4) -> (-40.55, -4)
  line L9 (-40.55, -4) -> (-40.55, -14)
  line L10 (-40.55, -14) -> (-28.55, -14)
  line L11 (-28.55, -14) -> (-28.55, -4)
  dimension "d23" = 57.1
  dimension "d24" = 12
  dimension "d25" = 10
  dimension "d26" = 12
  constraint horizontal L4
  constraint vertical L5
  constraint horizontal L6
  constraint vertical L7
  constraint coincident L2.end L3.start
  constraint horizontal L8
  constraint vertical L9
  constraint horizontal L10
  constraint vertical L11
  constraint horizontal L6.end L10.end
  constraint horizontal L2.end L8.start
  measures "d23" distance of L2.end L8.start
  measures "d24" distance of L5 L7
  measures "d25" distance of L4 L6
  measures "d26" distance of L9 L11
extrude "Extrude5" add sketch "Sketch6" against normal blind 20 contours L3 L4 L5 L6 L7 | L8 L9 L10 L11 bodies 1
sketch "Sketch7" plane through (0, 0, -4) normal (0, 0, 1) x (-1, 0, 0)
  line L0 (-30.55, -20) -> (-30.55, 0)
  line L1 (-30.55, 0) -> (-40.55, 0)
  line L2 (-40.55, 0) -> (-40.55, -20)
  line L3 (-40.55, -20) -> (-30.55, -20)
  line L4 (40.55, 0) -> (40.55, -20)
  point P0 (-34.75, -10)
  point P1 (34.75, -10)
  dimension "d29" = 5.8
  dimension "d30" = 5.8
  dimension "d31" = 10
  constraint horizontal P0 P1
  measures "d29" distance of L2 P0
  measures "d30" distance of P1 L4
  measures "d31" distance of L1 P0
hole "Hole1" at (34.75, 10, -4) at (-34.75, 10, -4) direction (0, 0, -1) diameter 5.3 depth 20 tip angle 180 counterbore diameter 10 counterbore depth 5 bodies 1
fillet "Fillet1" radius 2 2 edges at (40.55, 20, -9) (-40.55, 20, -9) on bodies 1
fillet "Fillet2" radius 2 4 edges at (30.55, 57, 10) (-30.55, 57, 10) (29.55, 20, 0) (-29.55, 20, 0) on bodies 1
sketch "Sketch8" plane through (0, 0, 0) normal (0, -1, 0) x (1, 0, 0)
  line L0 (30.55, -4) -> (30.55, 20)
  line L1 (30.55, 20) -> (28.55, 20)
  line L2 (28.55, 20) -> (28.55, -14)
  line L3 (28.55, -14) -> (40.55, -14)
  line L4 (40.55, -14) -> (40.55, -4)
  line L5 (40.55, -4) -> (30.55, -4)
  line L6 (30.55, 20) -> (28.55, 20)
  line L7 (30.55, 36.5) -> (30.55, 20)
  line L8 (-30.55, 20) -> (-28.55, 20)
  line L9 (-30.55, 36.5) -> (-30.55, 20)
  line L10 (28.55, 20) -> (-28.55, 20)
  line L11 (-19.3, 36.5) -> (-19.3, 34.25)
  line L12 (-24.3, 29.25) -> (-26.05, 29.25)
  line L13 (19.3, 36.5) -> (19.3, 34.25)
  line L14 (24.3, 29.25) -> (26.05, 29.25)
  line L15 (-28.55, 26.75) -> (-28.55, 20)
  line L16 (28.55, 26.75) -> (28.55, 20)
  line L17 (-28.05, 39) -> (-21.8, 39)
  line L18 (21.8, 39) -> (28.05, 39)
  arc A0 (30.55, 36.5) -> (28.05, 39) centre (28.05, 36.5) ccw
  arc A1 (-28.05, 39) -> (-30.55, 36.5) centre (-28.05, 36.5) ccw
  arc A2 (21.8, 39) -> (19.3, 36.5) centre (21.8, 36.5) ccw
  arc A3 (28.55, 26.75) -> (26.05, 29.25) centre (26.05, 26.75) ccw
  arc A4 (-26.05, 29.25) -> (-28.55, 26.75) centre (-26.05, 26.75) ccw
  arc A5 (-19.3, 36.5) -> (-21.8, 39) centre (-21.8, 36.5) ccw
  arc A6 (19.3, 34.25) -> (24.3, 29.25) centre (24.3, 34.25) ccw
  arc A7 (-24.3, 29.25) -> (-19.3, 34.25) centre (-24.3, 34.25) ccw
  point P0 (-30.55, 39)
  point P1 (-19.3, 39)
  point P2 (-19.3, 29.25)
  point P3 (-28.55, 29.25)
  point P4 (19.3, 39)
  point P5 (19.3, 29.25)
  point P6 (28.55, 29.25)
  dimension "d41" = 61.1
  dimension "d51" = 9.75
  dimension "d52" = 9.75
  dimension "d53" = 9.25
  dimension "d54" = 9.25
  dimension "d55" = 11.25
  dimension "d56" = 9.25
  dimension "d57" = 2.5
  dimension "d58" = 2.5
  dimension "d59" = 5
  constraint horizontal L6
  constraint vertical L7
  constraint coincident L0.end L1.start
  constraint horizontal L8
  constraint vertical L9
  constraint horizontal L0.end L8.start
  constraint vertical L11
  constraint horizontal L12
  constraint vertical L13
  constraint horizontal L14
  constraint perpendicular L10 L15
  constraint coincident L1.end L2.start
  constraint perpendicular L6 L16
  constraint perpendicular L11 L17
  constraint horizontal P2 P5
  constraint tangent L18 A0
  constraint tangent L7 A0
  constraint coincident P0 L17
  constraint coincident P0 L9
  constraint tangent L17 A1
  constraint tangent L9 A1
  constraint equal A0 A1
  constraint coincident P4 L13
  constraint coincident P4 L18
  constraint tangent L13 A2
  constraint tangent L18 A2
  constraint coincident P6 L14
  constraint coincident P6 L16
  constraint tangent L14 A3
  constraint tangent L16 A3
  constraint equal A2 A3
  constraint coincident P3 L12
  constraint coincident P3 L15
  constraint tangent L12 A4
  constraint tangent L15 A4
  constraint equal A2 A4
  constraint coincident P1 L11
  constraint coincident P1 L17
  constraint tangent L11 A5
  constraint tangent L17 A5
  constraint equal A2 A5
  constraint coincident P5 L14
  constraint coincident P5 L13
  constraint tangent L14 A6
  constraint tangent L13 A6
  constraint coincident P2 L12
  constraint coincident P2 L11
  constraint tangent L12 A7
  constraint tangent L11 A7
  constraint equal A6 A7
  measures "d41" distance of L0.end L8.start
  measures "d51" distance of P1 P2
  measures "d52" distance of P4 P5
  measures "d53" distance of P2 P3
  measures "d54" distance of P5 P6
  measures "d55" distance of P0 P1
  measures "d56" distance of P6 L1.end
  measures "d57" radius of A0
  measures "d58" radius of A2
  measures "d59" radius of A6
extrude "Extrude6" add sketch "Sketch8" against normal blind 20 contours L1 L6 L7 L13 L14 L16 L18 A0 A2 A3 A6 | L8 L9 L11 L12 L15 L17 A1 A4 A5 A7 bodies 1
sketch "Sketch9" plane through (0, 20, 0) normal (0, 1, 0) x (-1, 0, 0)
  arc A0 (-19.3, 36.5) -> (-21.8, 39) centre (-21.8, 36.5) ccw
  line L0 (-21.8, 39) -> (-28.05, 39)
  arc A1 (-28.05, 39) -> (-30.55, 36.5) centre (-28.05, 36.5) ccw
  line L1 (-30.55, 36.5) -> (-30.55, 20)
  line L2 (-30.55, 20) -> (-28.55, 20)
  line L3 (-28.55, 20) -> (-28.55, 26.75)
  arc A2 (-26.05, 29.25) -> (-28.55, 26.75) centre (-26.05, 26.75) ccw
  line L4 (-26.05, 29.25) -> (-24.3, 29.25)
  arc A3 (-24.3, 29.25) -> (-19.3, 34.25) centre (-24.3, 34.25) ccw
  line L5 (-19.3, 34.25) -> (-19.3, 36.5)
  line L6 (30.55, 20) -> (30.55, 36.5)
  point P0 (-24.05, 34.05)
  point P1 (24.05, 34.05)
  dimension "d62" = 6.5
  dimension "d63" = 6.5
  dimension "d64" = 4.95
  constraint horizontal P0 P1
  measures "d62" distance of L1 P0
  measures "d63" distance of P1 L6
  measures "d64" distance of L0 P0
hole "Hole3" at (24.05, 20, 34.05) at (-24.05, 20, 34.05) direction (0, -1, 0) diameter 6.5 depth 12.5 tip angle 180 bodies 1
sketch "Sketch10" plane through (0, 7.5, 0) normal (0, 1, 0) x (-1, 0, 0)
  circle A0 centre (-24.05, 34.05) radius 3.25
  line L0 (-30.55, 36.5) -> (-30.55, 20)
  line L1 (30.55, 20) -> (30.55, 36.5)
  line L2 (-21.8, 39) -> (-28.05, 39)
  point P0 (-24.05, 34.05)
  point P1 (24.05, 34.05)
  dimension "d73" = 6.5
  dimension "d74" = 6.5
  dimension "d75" = 4.95
  constraint horizontal P0 P1
  measures "d73" distance of P0 L0
  measures "d74" distance of P1 L1
  measures "d75" distance of P0 L2
hole "Hole4" at (24.05, 7.5, 34.05) at (-24.05, 7.5, 34.05) direction (0, -1, 0) diameter 3.6 end through all counterbore diameter 6.5 counterbore depth 3 bodies 1
sketch "Sketch11" plane through (30.55, 0, 0) normal (1, 0, 0) x (0, 1, 0)
  line L0 (55.4221, 0) -> (55.4221, 20)
  line L1 (55.4221, 20) -> (20, 20)
  line L2 (20, 20) -> (20, 36.5)
  line L3 (20, 36.5) -> (0, 36.5)
  line L4 (0, 36.5) -> (0, -4)
  line L5 (0, -4) -> (7.2871, -4)
  line L6 (7.2871, -4) -> (12.7129, -4)
  line L7 (12.7129, -4) -> (20, -4)
  line L8 (20, -4) -> (20, -2)
  arc A0 (22, 0) -> (20, -2) centre (22, -2) ccw
  line L9 (22, 0) -> (55.4221, 0)
  arc A1 (8.659, 10.728) -> (8.6579, 11.8018) centre (7.8148, 11.264) ccw
  line L10 (8.659, 10.728) -> (3.8443, 3.1449)
  line L11 (3.8432, 19.3505) -> (8.6579, 11.8018)
  line L12 (0.0001, 38.0402) -> (0.0001, -4.0098)
  arc A2 (3.8432, 19.3505) -> (2.0001, 18.8128) centre (3.0001, 18.8128) ccw
  arc A3 (2.0001, 3.6809) -> (3.8443, 3.1449) centre (3.0001, 3.6809) ccw
  arc A4 (18.0001, 18.8128) -> (16.157, 19.3505) centre (17.0001, 18.8128) ccw
  line L13 (16.088, 21.9584) -> (10.853, 13.6232)
  line L14 (9.1559, 13.6286) -> (3.9952, 21.9638)
  line L15 (3.99, 0.515) -> (9.1549, 8.8941)
  line L16 (15.2412, 23.4902) -> (4.8454, 23.4902)
  line L17 (2.0001, 18.8128) -> (2.0001, 3.6809)
  arc A5 (10.8541, 8.8995) -> (9.1549, 8.8941) centre (10.0062, 8.3693) ccw
  line L18 (20.0001, 40.5402) -> (0.0001, 40.5402)
  arc A6 (3.99, 0.515) -> (4.8412, -1.0098) centre (4.8412, -0.0098) ccw
  line L19 (20.0001, 38.0402) -> (0.0001, 38.0402)
  arc A7 (4.8454, 23.4902) -> (3.9952, 21.9638) centre (4.8454, 22.4902) ccw
  line L20 (15.2454, -1.0098) -> (4.8412, -1.0098)
  line L21 (18.0001, 18.8128) -> (18.0001, 3.6809)
  arc A8 (16.088, 21.9584) -> (15.2412, 23.4902) centre (15.2412, 22.4902) ccw
  line L22 (16.1559, 3.1449) -> (11.3412, 10.728)
  arc A9 (9.1559, 13.6286) -> (10.853, 13.6232) centre (10.0062, 14.1551) ccw
  line L23 (10.8541, 8.8995) -> (16.0933, 0.5204)
  line L24 (11.3423, 11.8018) -> (16.157, 19.3505)
  arc A10 (11.3423, 11.8018) -> (11.3412, 10.728) centre (12.1854, 11.264) ccw
  line L25 (12.713, -4.0098) -> (20.0001, -4.0098)
  arc A11 (16.1559, 3.1449) -> (18.0001, 3.6809) centre (17.0001, 3.6809) ccw
  arc A12 (15.2454, -1.0098) -> (16.0933, 0.5204) centre (15.2454, -0.0098) ccw
  line L26 (0.0001, -4.0098) -> (7.2872, -4.0098)
  line L27 (20.0001, -4.0098) -> (20.0001, 38.0402)
  point P0 (9.0001, 11.2652)
  point P1 (11.0001, 11.2652)
  point P2 (18.0001, 0.2402)
  point P3 (2.0001, 22.2402)
  point P4 (10.0001, 10.2652)
  point P5 (10.0501, 11.2402)
  point P6 (17.0501, 23.4902)
  point P7 (2.0001, 0.2402)
  point P8 (3.0501, -1.0098)
  point P9 (17.0501, -1.0098)
  point P10 (3.0501, 23.4902)
  point P11 (10.0001, 12.2652)
  point P12 (0.0001, 12.2652)
  point P13 (18.0001, 22.2402)
  dimension "d80" = 3
  dimension "d81" = 17.05
  dimension "d82" = 2
  dimension "d83" = 2
  dimension "d86" = 22
  dimension "d87" = 22
  dimension "d88" = 14
  dimension "d89" = 14
  dimension "d90" = 4.25
  dimension "d91" = 3.05
  dimension "d92" = 1
  constraint perpendicular L16 L27
  constraint perpendicular L16 L17
  constraint coincident P6 L13
  constraint coincident P6 L16
  constraint tangent L13 A8
  constraint tangent L16 A8
  constraint coincident P10 L16
  constraint coincident P10 L14
  constraint tangent L16 A7
  constraint tangent L14 A7
  constraint equal A7 A8
  constraint tangent L14 A9
  constraint tangent L13 A9
  constraint equal A8 A9
  constraint tangent A1 L11
  constraint tangent A1 L10
  constraint equal A1 A8
  constraint coincident P7 L10
  constraint coincident P7 L17
  constraint tangent L10 A3
  constraint tangent A3 L17
  constraint equal A3 A8
  constraint coincident P3 L17
  constraint coincident P3 L11
  constraint tangent A2 L17
  constraint tangent L11 A2
  constraint equal A2 A8
  constraint coincident P8 L15
  constraint coincident P8 L20
  constraint tangent L15 A6
  constraint tangent A6 L20
  constraint equal A6 A8
  constraint coincident P9 L20
  constraint coincident P9 L23
  constraint tangent L20 A12
  constraint tangent L23 A12
  constraint equal A8 A12
  constraint coincident P2 L22
  constraint coincident P2 L21
  constraint tangent L22 A11
  constraint tangent L21 A11
  constraint equal A8 A11
  constraint coincident P13 L24
  constraint coincident P13 L21
  constraint tangent A4 L24
  constraint tangent A4 L21
  constraint equal A4 A8
  constraint tangent L22 A10
  constraint tangent L24 A10
  constraint equal A8 A10
  constraint tangent L15 A5
  constraint tangent A5 L23
  constraint equal A5 A8
  measures "d80" distance of L20 L25
  measures "d81" distance of L16 L18
  measures "d82" distance of L21 L27
  measures "d83" distance of L12 L17
  measures "d86" distance of P2 P13
  measures "d87" distance of P3 P7
  measures "d88" distance of P8 P9
  measures "d89" distance of P6 P10
  measures "d90" distance of P2 L25
  measures "d91" distance of P8 L12
  measures "d92" radius of A8
extrude "Extrude7" cut sketch "Sketch11" against normal blind 65 contours A1 L10 L11 A2 A3 L17 | A4 L21 L22 L24 A10 A11 | L13 L14 L16 A7 A8 A9 | L15 A5 A6 L20 L23 A12 bodies 1